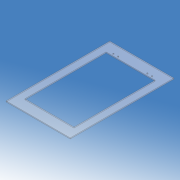
# Autodesk Inventor part: NASA-20-EBOX-T2-01
Saved by Autodesk Inventor 2020 (Build 240168000, 168)
## iProperties
Created: 2019-09-23
Part Number: NASA-20-EBOX-T2-01
Material: Polycarbonate, Clear
Document SubType Name: Modeling
Designer: mpark
Density: 1.2 g/cm^3
Appearance: Polycarbonate - Clear
Author: mpark
Autodesk Inventor part; units mm, degrees
ref_plane "YZ Plane" through (0, 0, 0) normal (1, 0, 0) x (0, 1, 0)
ref_plane "XZ Plane" through (0, 0, 0) normal (0, 1, 0) x (-1, 0, 0)
ref_plane "XY Plane" through (0, 0, 0) normal (0, 0, 1) x (1, 0, 0)
sketch "Sketch1" plane through (0, 0, 0) normal (0, 1, 0) x (-1, 0, 0)
  line L0 (107.95, -174.625) -> (-107.95, -174.625)
  line L1 (-107.95, -174.625) -> (-107.95, 174.625)
  line L2 (-107.95, 174.625) -> (107.95, 174.625)
  line L3 (107.95, 174.625) -> (107.95, -174.625)
  line L4 (107.95, -174.625) -> (-107.95, 174.625) construction
  line L5 (-107.95, -174.625) -> (107.95, 174.625) construction
  point P0 (0, 0)
  dimension "d0" = 215.9
  dimension "d1" = 349.25
  constraints: 12 end point, 2 midpoint, 2 parallel, 1 horizontal, 1 perpendicular
  measures "d0" distance of L1.end L2.end
  measures "d1" distance of L0.end L1.end
extrude "Thickness" add sketch "Sketch1" along normal blind 3.175
sketch "Cutout Sketch" plane through (0, 3.175, 0) normal (0, 1, 0) x (1, 0, 0)
  line L0 (107.95, -174.625) -> (107.95, 174.625) projected
  line L1 (107.95, 174.625) -> (-107.95, 174.625) projected
  line L2 (-107.95, 174.625) -> (-107.95, -174.625) projected
  line L3 (-107.95, -174.625) -> (107.95, -174.625) projected
  line L4 (-82.55, 136.525) -> (82.55, 136.525)
  line L5 (82.55, 136.525) -> (82.55, -136.525)
  line L6 (82.55, -136.525) -> (-82.55, -136.525)
  line L7 (-82.55, -136.525) -> (-82.55, 136.525)
  point P0 (0, 0)
  dimension "d4" = 25.4
  dimension "d5" = 38.1
  dimension "d8" = 38.1
  dimension "d9" = 25.4
  constraints: 8 end point, 2 parallel, 1 horizontal, 1 perpendicular
  measures "d4" distance between parallel lines of L7 L2
  measures "d5" distance between parallel lines of L1 L4
  measures "d8" distance between parallel lines of L3 L6
  measures "d9" distance between parallel lines of L0 L5
extrude "Cutout" cut sketch "Cutout Sketch" against normal blind 25.4 contours L4 L5 L6 L7
sketch "Sketch3" plane through (0, 3.175, 0) normal (0, 1, 0) x (1, 0, 0)
  line L0 (44.45, 149.225) -> (44.45, 137.9537) projected
  line L1 (44.45, 137.9537) -> (49.1744, 137.9537) projected
  line L2 (49.1744, 137.9537) -> (49.1744, 136.525) projected
  line L3 (49.1744, 136.525) -> (54.737, 136.525) projected
  line L4 (54.737, 136.525) -> (54.737, 137.9537) projected
  line L5 (54.737, 137.9537) -> (59.563, 137.9537) projected
  line L6 (59.563, 137.9537) -> (59.563, 136.525) projected
  line L7 (59.563, 136.525) -> (65.1256, 136.525) projected
  line L8 (65.1256, 136.525) -> (65.1256, 137.9537) projected
  line L9 (65.1256, 137.9537) -> (69.85, 137.9537) projected
  line L10 (69.85, 149.225) -> (69.85, 137.9537) projected
  line L11 (44.45, 149.225) -> (69.85, 149.225) projected
  circle A0 centre (65.0875, 144.0656) radius 2.0955 projected
  circle A1 centre (49.2125, 144.0656) radius 2.0955 projected
  line L12 (-69.85, 149.225) -> (-69.85, 137.9537) projected
  line L13 (-69.85, 137.9537) -> (-65.1256, 137.9537) projected
  line L14 (-65.1256, 137.9537) -> (-65.1256, 136.525) projected
  line L15 (-65.1256, 136.525) -> (-59.563, 136.525) projected
  line L16 (-59.563, 136.525) -> (-59.563, 137.9537) projected
  line L17 (-59.563, 137.9537) -> (-54.737, 137.9537) projected
  line L18 (-54.737, 137.9537) -> (-54.737, 136.525) projected
  line L19 (-54.737, 136.525) -> (-49.1744, 136.525) projected
  line L20 (-49.1744, 136.525) -> (-49.1744, 137.9537) projected
  line L21 (-49.1744, 137.9537) -> (-44.45, 137.9537) projected
  line L22 (-44.45, 149.225) -> (-44.45, 137.9537) projected
  line L23 (-69.85, 149.225) -> (-44.45, 149.225) projected
  circle A2 centre (-49.2125, 144.0656) radius 2.0955 projected
  circle A3 centre (-65.0875, 144.0656) radius 2.0955 projected
  point P0 (0, 0)
hole "Hole1" at (65.0875, 3.175, -144.0656) at (49.2125, 3.175, -144.0656) at (-65.0875, 3.175, -144.0656) at (-49.2125, 3.175, -144.0656) direction (0, -1, 0) diameter 3.5 depth 2
body "Solid1"
